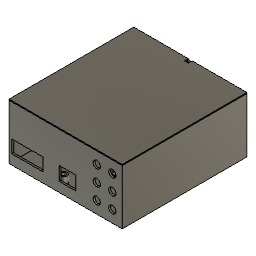
Case (Autodesk Fusion 360 design; units mm, degrees)
Autodesk Fusion 360 part; units mm, degrees
note: some values were not read from the file. Chosen so that the rebuilt part matches the saved one: which bodies a step acts on; which face or edge a step refers to. Set by a fixed rule: which sketch regions a step uses.
sketch "Base" plane through (0, 0, 0) normal (0, 0, 1) x (1, 0, 0) in component "PCB"
  line L0 (58.9, 60.9) -> (0, 60.9)
  line L1 (0, 60.9) -> (0, 0)
  line L2 (0, 0) -> (58.9, 0)
  line L3 (58.9, 0) -> (58.9, 60.9)
  circle A0 centre (3.45, 57.45) radius 1.6
  line L4 (29.45, 60.9) -> (29.45, 0) construction
  line L5 (0, 30.45) -> (58.9, 30.45) construction
  circle A1 centre (55.45, 57.45) radius 1.6
  circle A2 centre (3.45, 3.45) radius 1.6
  circle A3 centre (55.45, 3.45) radius 1.6
  dimension "d1" = 58.9
  dimension "d2" = 60.9
  dimension "d3" = 3.2
  dimension "d4" = 3.45
  dimension "d5" = 3.45
  constraint horizontal L0
  constraint vertical L1
  constraint horizontal L2
  constraint vertical L3
  constraint coincident L1.end L2.start
  constraint midpoint L0 L4.start
  constraint midpoint L2 L4.end
  constraint midpoint L1 L5.start
  constraint midpoint L3 L5.end
  constraint symmetric A0 L4 A1
  constraint symmetric A0 L5 A2
  constraint symmetric L5 A1 A3
  measures "d1" distance of L1.end L2.end
  measures "d2" distance of L0.end L1.end
  measures "d3" diameter of A0
  measures "d4" distance of L0 A0.centre
  measures "d5" distance of L1 A0.centre
extrude "Extrude1" add sketch "Base" along normal blind 24.2 makes body 1 in component "PCB"
sketch "USB port" plane through (0, 60.9, 0) normal (0, 1, 0) x (-1, 0, 0) in component "PCB"
  line L0 (-58.9, 0) -> (0, 0)
  line L1 (0, 0) -> (0, 24.2)
  line L2 (0, 24.2) -> (-58.9, 24.2)
  line L3 (-58.9, 24.2) -> (-58.9, 0)
  line L4 (-44.9, 16.5) -> (-36.9, 16.5)
  line L5 (-36.9, 16.5) -> (-36.9, 13.5)
  line L6 (-36.9, 13.5) -> (-44.9, 13.5)
  line L7 (-44.9, 13.5) -> (-44.9, 16.5)
  dimension "d8" = 8
  dimension "d9" = 3
  dimension "d10" = 14
  dimension "d11" = 13.5
  constraint horizontal L4
  constraint vertical L5
  constraint horizontal L6
  constraint vertical L7
  measures "d8" distance of L4.start L4.end
  measures "d9" distance of L4.start L6.end
  measures "d10" distance of L3 L7
  measures "d11" distance of L0 L6
extrude "Extrude2" add sketch "USB port" along normal blind 1 contours L4 L5 L6 L7 bodies 1 in component "PCB"
sketch "Base (2)" plane through (0, 0, 0) normal (0, 0, 1) x (1, 0, 0) in component "RJ45 breakout"
  line L0 (35.9, 21.4) -> (0, 21.4)
  line L1 (0, 21.4) -> (0, 0)
  line L2 (0, 0) -> (35.9, 0)
  line L3 (35.9, 0) -> (35.9, 21.4)
  circle A0 centre (4, 5) radius 1.6
  line L4 (17.95, 21.4) -> (17.95, 0) construction
  circle A1 centre (31.9, 5) radius 1.6
  dimension "d14" = 35.9
  dimension "d15" = 21.4
  dimension "d16" = 3.2
  dimension "d17" = 5
  dimension "d18" = 4
  constraint horizontal L0
  constraint vertical L1
  constraint horizontal L2
  constraint vertical L3
  constraint coincident L1.end L2.start
  constraint midpoint L0 L4.start
  constraint midpoint L2 L4.end
  constraint symmetric A0 L4 A1
  measures "d14" distance of L0.start L0.end
  measures "d15" distance of L0.end L1.end
  measures "d16" diameter of A0
  measures "d17" distance of L2 A0.centre
  measures "d18" distance of L1 A0.centre
extrude "Extrude1'" add sketch "Base (2)" along normal blind 1.5 separate body makes body 2 in component "RJ45 breakout"
sketch "Port" plane through (0, 0, 1.5) normal (0, 0, 1) x (-1, 0, 0) in component "RJ45 breakout"
  circle A0 centre (-31.9, -5) radius 1.6
  circle A1 centre (-4, -5) radius 1.6
  line L0 (-35.9, 0) -> (-35.9, -21.4)
  line L1 (-35.9, -21.4) -> (0, -21.4)
  line L2 (0, -21.4) -> (0, 0)
  line L3 (0, 0) -> (-35.9, 0)
  line L4 (-9.8, -13.3) -> (-26.1, -13.3)
  line L5 (-26.1, -13.3) -> (-26.1, 2.1)
  line L6 (-26.1, 2.1) -> (-9.8, 2.1)
  line L7 (-9.8, 2.1) -> (-9.8, -13.3)
  dimension "d21" = 16.3
  dimension "d22" = 15.4
  dimension "d23" = 2.1
  dimension "d24" = 35.9
  dimension "d25" = 9.8
  constraint horizontal L4
  constraint vertical L5
  constraint horizontal L6
  constraint vertical L7
  measures "d21" distance of L4.start L4.end
  measures "d22" distance of L4.start L6.end
  measures "d23" distance of L3 L6
  measures "d24" distance of L0.end L1.end
  measures "d25" distance of L2 L7
extrude "Extrude2'" add sketch "Port" along normal blind 13.3 contours L3 L5 L6 L7 | L3 L4 L5 L7 bodies 2 in component "RJ45 breakout"
sketch "Base (3)" plane through (0, 0, 0) normal (0, 0, 1) x (1, 0, 0) in component "UART to RS-232 converter"
  line L0 (31.6, 28) -> (0, 28)
  line L1 (0, 28) -> (0, 0)
  line L2 (0, 0) -> (31.6, 0)
  line L3 (31.6, 0) -> (31.6, 28)
  circle A0 centre (2.1, 25.7) radius 1.6
  line L4 (15.8, 28) -> (15.8, 0) construction
  circle A1 centre (29.5, 25.7) radius 1.6
  dimension "d28" = 28
  dimension "d29" = 31.6
  dimension "d30" = 3.2
  dimension "d31" = 2.1
  dimension "d32" = 2.3
  constraint horizontal L0
  constraint vertical L1
  constraint horizontal L2
  constraint vertical L3
  constraint coincident L1.end L2.start
  constraint midpoint L0 L4.start
  constraint midpoint L2 L4.end
  constraint symmetric A0 L4 A1
  measures "d28" distance of L0.end L1.end
  measures "d29" distance of L0.start L0.end
  measures "d30" diameter of A0
  measures "d31" distance of L1 A0.centre
  measures "d32" distance of L0 A0.centre
extrude "Extrude1''" add sketch "Base (3)" along normal blind 1.5 separate body makes body 3 in component "UART to RS-232 converter"
sketch "Port (2)" plane through (0, 0, 1.5) normal (0, 0, 1) x (-1, 0, 0) in component "UART to RS-232 converter"
  circle A0 centre (-29.5, -25.7) radius 1.6
  circle A1 centre (-2.1, -25.7) radius 1.6
  line L0 (-31.6, 0) -> (-31.6, -28)
  line L1 (-31.6, -28) -> (0, -28)
  line L2 (0, -28) -> (0, 0)
  line L3 (0, 0) -> (-31.6, 0)
  line L4 (0, -12.3) -> (-31.6, -12.3)
  line L5 (-31.6, -12.3) -> (-31.6, 17.9)
  line L6 (-31.6, 17.9) -> (0, 17.9)
  line L7 (0, 17.9) -> (0, -12.3)
  dimension "d35" = 30.2
  dimension "d36" = 12.3
  constraint horizontal L4
  constraint vertical L5
  constraint horizontal L6
  constraint vertical L7
  constraint collinear L2 L7
  constraint collinear L0 L5
  measures "d35" distance of L4.start L6.end
  measures "d36" distance of L3 L4
extrude "Extrude2''" add sketch "Port (2)" along normal blind 12.7 contours L0 L2 L3 L4 L5 L7 | L3 L5 L6 L7 bodies 3 in component "UART to RS-232 converter"
sketch "Sketch1" plane through (0, 0, 0) normal (0, 0, 1) x (1, 0, 0) in component "Relay"
  line L0 (16.35, -19.7) -> (-16.35, -19.7)
  line L1 (-16.35, -19.7) -> (-16.35, 19.7)
  line L2 (-16.35, 19.7) -> (16.35, 19.7)
  line L3 (16.35, 19.7) -> (16.35, -19.7)
  line L4 (16.35, -19.7) -> (-16.35, 19.7) construction
  line L5 (-16.35, -19.7) -> (16.35, 19.7) construction
  dimension "d139" = 32.7
  dimension "d140" = 39.4
  constraint horizontal L0
  constraint perpendicular L0 L1
  constraint parallel L0 L2
  constraint parallel L1 L3
  constraint coincident L4 origin
  constraint coincident L5 origin
  measures "d139" distance of L1.end L2.end
  measures "d140" distance of L0.start L2.end
extrude "Extrude1'''" add sketch "Sketch1" along normal blind 21 separate body makes body 4 in component "Relay"
ref_plane "WorkPlane1" through (0, 0, 10.5) normal (-1, 0, 0) x (0, -1, 0) in component "Relay"
ref_plane "WorkPlane2" through (0, 0, 10.5) normal (0, -1, 0) x (1, 0, 0) in component "Relay"
sketch "Sketch2" plane through (0, 0, 21) normal (0, 0, 1) x (-1, 0, 0) in component "Relay"
  line L0 (-16.35, -19.7) -> (16.35, -19.7)
  line L1 (16.35, -19.7) -> (16.35, 19.7)
  line L2 (16.35, 19.7) -> (-16.35, 19.7)
  line L3 (-16.35, 19.7) -> (-16.35, -19.7)
  circle A0 centre (12.55, -15.7) radius 1.5
  line L4 (0, -23.64) -> (0, 23.64)
  circle A1 centre (-12.55, -15.7) radius 1.5
  line L5 (19.62, 0) -> (-19.62, 0)
  circle A2 centre (12.55, 15.7) radius 1.5
  circle A3 centre (-12.55, 15.7) radius 1.5
  dimension "d143" = 3
  dimension "d144" = 4
  dimension "d145" = 3.8
  constraint symmetric A0 L4 A1
  constraint symmetric A0 L5 A2
  constraint symmetric A1 L5 A3
  measures "d143" diameter of A0
  measures "d144" distance of L0 A0.centre
  measures "d145" distance of L1 A0.centre
extrude "Extrude2'''" cut sketch "Sketch2" against normal up to surface (21 mm away) contours A0 | A1 | A2 | A3 bodies 4 in component "Relay"
sketch "Sketch1 (2)" plane through (0, 0, 0) normal (0, 1, 0) x (1, 0, 0) in component "Banana socket"
  circle A0 centre (0, 0) radius 6
  dimension "d148" = 12
  constraint coincident A0.centre origin
  measures "d148" diameter of A0
extrude "Extrude1''''" add sketch "Sketch1 (2)" along normal blind 24 separate body makes body 5 in component "Banana socket"
sketch "Sketch2 (2)" plane through (0, 24, 0) normal (0, 1, 0) x (-1, 0, 0) in component "Banana socket"
  circle A0 centre (0, 0) radius 6
  circle A1 centre (0, 0) radius 3.8
  dimension "d151" = 7.6
  constraint coincident A0.centre A1.centre
  measures "d151" diameter of A1
extrude "Extrude2''''" add sketch "Sketch2 (2)" along normal blind 21.5 contours A1 bodies 5 in component "Banana socket"
other "GeometricRelationship15"
other "GeometricRelationship18"
other "GeometricRelationship19"
pattern_linear "00000000-0000-0000-0000-000000000000" [suppressed]
sketch "Sketch10" plane through (0, 0, 0) normal (0, 0, 1) x (1, 0, 0) in component "Case"
  circle A0 centre (8.2, 75.65) radius 1.6
  circle A1 centre (60.2, 75.65) radius 1.6
  circle A2 centre (60.2, 21.65) radius 1.6
  circle A3 centre (8.2, 21.65) radius 1.6
  circle A4 centre (6.85, -7.6) radius 1.6
  circle A5 centre (34.25, -7.6) radius 1.6
  circle A6 centre (77.45, 15.7) radius 1.5
  circle A7 centre (102.55, 15.7) radius 1.5
  circle A8 centre (102.55, -15.7) radius 1.5
  circle A9 centre (77.45, -15.7) radius 1.5
  circle A10 centre (77.45, 65.1) radius 1.5
  circle A11 centre (102.55, 65.1) radius 1.5
  circle A12 centre (77.45, 33.7) radius 1.5
  circle A13 centre (102.55, 33.7) radius 1.5
  circle A14 centre (50.35, -44.1) radius 1.6
  circle A15 centre (78.25, -44.1) radius 1.6
  circle A16 centre (34.25, -7.6) radius 1.6
  circle A17 centre (6.85, -7.6) radius 1.6
  line L0 (36.35, -5.3) -> (36.35, -33.3)
  line L1 (36.35, -33.3) -> (4.75, -33.3)
  line L2 (4.75, -33.3) -> (4.75, -5.3)
  line L3 (4.75, -5.3) -> (36.35, -5.3)
  circle A18 centre (8.2, 75.65) radius 2
  circle A19 centre (8.2, 75.65) radius 3.5
  circle A20 centre (60.2, 75.65) radius 2
  circle A21 centre (60.2, 75.65) radius 3.5
  circle A22 centre (8.2, 21.65) radius 2
  circle A23 centre (8.2, 21.65) radius 3.5
  circle A24 centre (60.2, 21.65) radius 2
  circle A25 centre (60.2, 21.65) radius 3.5
  circle A26 centre (77.45, 65.1) radius 2
  circle A27 centre (77.45, 65.1) radius 3.5
  circle A28 centre (102.55, 65.1) radius 2
  circle A29 centre (102.55, 65.1) radius 3.5
  circle A30 centre (102.55, 33.7) radius 2
  circle A31 centre (102.55, 33.7) radius 3.5
  circle A32 centre (77.45, 33.7) radius 2
  circle A33 centre (77.45, 33.7) radius 3.5
  circle A34 centre (77.45, 15.7) radius 2
  circle A35 centre (77.45, 15.7) radius 3.5
  circle A36 centre (102.55, 15.7) radius 2
  circle A37 centre (102.55, 15.7) radius 3.5
  circle A38 centre (102.55, -15.7) radius 2
  circle A39 centre (102.55, -15.7) radius 3.5
  circle A40 centre (77.45, -15.7) radius 2
  circle A41 centre (77.45, -15.7) radius 3.5
  circle A42 centre (6.85, -7.6) radius 2
  circle A43 centre (6.85, -7.6) radius 3.5
  circle A44 centre (34.25, -7.6) radius 2
  circle A45 centre (34.25, -7.6) radius 3.5
  circle A46 centre (50.35, -44.1) radius 2
  circle A47 centre (50.35, -44.1) radius 3.5
  circle A48 centre (78.25, -44.1) radius 2
  circle A49 centre (78.25, -44.1) radius 3.5
  circle A50 centre (20.55, -30.8) radius 2.5
  point P0 (20.55, -33.3)
  dimension "d219" = 4
  dimension "d220" = 7
  dimension "d221" = 4
  dimension "d222" = 7
  dimension "d223" = 4
  dimension "d224" = 7
  dimension "d225" = 4
  dimension "d226" = 7
  dimension "d227" = 4
  dimension "d228" = 7
  dimension "d229" = 4
  dimension "d230" = 7
  dimension "d231" = 4
  dimension "d232" = 7
  dimension "d233" = 4
  dimension "d234" = 7
  dimension "d235" = 4
  dimension "d236" = 7
  dimension "d237" = 4
  dimension "d238" = 7
  dimension "d239" = 4
  dimension "d240" = 7
  dimension "d241" = 4
  dimension "d242" = 7
  dimension "d243" = 4
  dimension "d244" = 7
  dimension "d245" = 4
  dimension "d246" = 7
  dimension "d247" = 4
  dimension "d248" = 7
  dimension "d249" = 4
  dimension "d250" = 7
  dimension "d251" = 5
  constraint coincident A0.centre A18.centre
  constraint coincident A1.centre A20.centre
  constraint coincident A3.centre A22.centre
  constraint coincident A2.centre A24.centre
  constraint coincident A10.centre A26.centre
  constraint coincident A11.centre A28.centre
  constraint coincident A13.centre A30.centre
  constraint coincident A12.centre A32.centre
  constraint coincident A6.centre A34.centre
  constraint coincident A7.centre A36.centre
  constraint coincident A8.centre A38.centre
  constraint coincident A9.centre A40.centre
  constraint coincident A4.centre A17.centre
  constraint coincident A5.centre A16.centre
  constraint coincident A14.centre A46.centre
  constraint coincident A15.centre A48.centre
  constraint midpoint L1 P0
  constraint vertical A50.centre P0
  constraint tangent L1 A50
  measures "d219" diameter of A18
  measures "d220" diameter of A19
  measures "d221" diameter of A20
  measures "d222" diameter of A21
  measures "d223" diameter of A22
  measures "d224" diameter of A23
  measures "d225" diameter of A24
  measures "d226" diameter of A25
  measures "d227" diameter of A26
  measures "d228" diameter of A27
  measures "d229" diameter of A28
  measures "d230" diameter of A29
  measures "d231" diameter of A30
  measures "d232" diameter of A31
  measures "d233" diameter of A32
  measures "d234" diameter of A33
  measures "d235" diameter of A34
  measures "d236" diameter of A35
  measures "d237" diameter of A36
  measures "d238" diameter of A37
  measures "d239" diameter of A38
  measures "d240" diameter of A39
  measures "d241" diameter of A40
  measures "d242" diameter of A41
  measures "d243" diameter of A42
  measures "d244" diameter of A43
  measures "d245" diameter of A44
  measures "d246" diameter of A45
  measures "d247" diameter of A46
  measures "d248" diameter of A47
  measures "d249" diameter of A48
  measures "d250" diameter of A49
  measures "d251" diameter of A50
extrude "Extrude10" add sketch "Sketch10" against normal blind 8 separate body contours L0 L3 A45 | L0 L3 A45 | A50 | L2 L3 A43 | L2 L3 A43 | A19 | A21 | A23 | A25 | A27 | A29 | A31 | A33 | A35 | A37 | A39 | A41 | A47 | A49 makes body 6 at (23.0469, -30.9246, -5.3333) makes body 7 at (106.0456, -15.8745, -5.3333) makes body 8 at (106.0456, 33.5255, -5.3333) makes body 9 at (11.6956, 21.4755, -5.3333) makes body 10 at (57.2135, 73.825, -5.3333) makes body 11 at (100.1062, 62.5945, -5.3333) makes body 12 at (101.4353, 12.3823, -5.3333) makes body 13 at (37.7326, -7.2515, -2.6667) makes body 14 at (53.8456, -44.2745, -5.3333) makes body 15 at (76.3353, -19.0177, -5.3333) makes body 16 at (80.1312, 35.9498, -5.3333) makes body 17 at (63.6956, 21.4755, -5.3333) makes body 18 at (5.2135, 73.825, -5.3333) makes body 19 at (80.9456, 64.9255, -5.3333) makes body 20 at (80.9456, 15.5255, -5.3333) makes body 21 at (10.3456, -7.7745, -5.3333) makes body 22 at (75.8062, -46.6055, -5.3333) in component "Case"
sketch "Sketch11" plane through (0, 0, -8) normal (0, 0, -1) x (1, 0, 0) in component "Case"
  circle A0 centre (34.25, 7.6) radius 2
  circle A1 centre (34.25, 7.6) radius 3.5
  circle A2 centre (8.2, -75.65) radius 1.6
  circle A3 centre (8.2, -21.65) radius 1.6
  circle A4 centre (60.2, -21.65) radius 1.6
  circle A5 centre (60.2, -75.65) radius 1.6
  line L0 (63.65, -79.1) -> (63.65, -18.2)
  line L1 (63.65, -18.2) -> (4.75, -18.2)
  line L2 (4.75, -18.2) -> (4.75, -79.1)
  line L3 (4.75, -79.1) -> (63.65, -79.1)
  line L4 (109.45, 32.7) -> (117.05, 32.7)
  line L5 (117.05, 54.2) -> (109.45, 54.2)
  line L6 (2.35, 52.2) -> (122.05, 52.2)
  line L7 (122.05, 52.2) -> (122.05, -80.1)
  line L8 (122.05, -80.1) -> (2.35, -80.1)
  line L9 (2.35, -80.1) -> (2.35, 52.2)
  circle A6 centre (6.85, 7.6) radius 3.5
  line L10 (56.15, 51.2) -> (72.45, 51.2)
  line L11 (72.45, 51.2) -> (72.45, 35.8)
  line L12 (72.45, 35.8) -> (56.15, 35.8)
  line L13 (56.15, 35.8) -> (56.15, 51.2)
  dimension "d255" = 1
  dimension "d256" = 5
  dimension "d257" = 4.5
  dimension "d258" = 7
  dimension "d264" = 1
  constraint horizontal L6
  constraint vertical L7
  constraint horizontal L8
  constraint vertical L9
  measures "d255" distance of L3 L8
  measures "d256" distance of L4.end L7
  measures "d257" distance of L9 A6.centre
  measures "d258" diameter of A6
  measures "d264" distance of L6 L10
extrude "Extrude11" add sketch "Sketch11" along normal blind 2 contours A0 | A1 | A2 | A3 | A4 | A5 | L0 L1 L2 L3 | L6 L7 L8 L9 | A6 | L10 L11 L12 L13 bodies 6 7 8 9 10 11 12 13 14 15 16 17 18 19 20 21 22 in component "Case"
sketch "Sketch12" plane through (0, 0, -10) normal (0, 0, -1) x (1, 0, 0) in component "Case"
  line L0 (2.35, -80.1) -> (122.05, -80.1)
  line L1 (122.05, -80.1) -> (122.05, 52.2)
  line L2 (122.05, 52.2) -> (2.35, 52.2)
  line L3 (2.35, 52.2) -> (2.35, -80.1)
  line L4 (0.35, -82.1) -> (124.05, -82.1)
  line L5 (124.05, -82.1) -> (124.05, 54.2)
  line L6 (124.05, 54.2) -> (0.35, 54.2)
  line L7 (0.35, 54.2) -> (0.35, -82.1)
  dimension "d261" = 2
extrude "Extrude12" add sketch "Sketch12" against normal blind 60 bodies 6 in component "Case"
sketch "Sketch13" plane through (0, 82.1, 0) normal (0, 1, 0) x (-1, 0, 0) in component "Case"
  line L0 (-124.05, -10) -> (-0.35, -10)
  line L1 (-0.35, -10) -> (-0.35, 50)
  line L2 (-0.35, 50) -> (-124.05, 50)
  line L3 (-124.05, 50) -> (-124.05, -10)
  line L4 (-49.65, 13.5) -> (-41.65, 13.5)
  line L5 (-41.65, 13.5) -> (-41.65, 16.5)
  line L6 (-41.65, 16.5) -> (-49.65, 16.5)
  line L7 (-49.65, 16.5) -> (-49.65, 13.5)
  line L8 (-51.65, 19.5) -> (-39.65, 19.5)
  line L9 (-39.65, 19.5) -> (-39.65, 10.5)
  line L10 (-39.65, 10.5) -> (-51.65, 10.5)
  line L11 (-51.65, 10.5) -> (-51.65, 19.5)
  dimension "d265" = 12
  dimension "d266" = 9
  dimension "d267" = 3
  dimension "d268" = 8
  dimension "d269" = 2
  dimension "d270" = 3
  constraint horizontal L8
  constraint vertical L9
  constraint horizontal L10
  constraint vertical L11
  measures "d265" distance of L8.start L8.end
  measures "d266" distance of L8.end L9.end
  measures "d267" distance of L4.start L6.end
  measures "d268" distance of L4.start L4.end
  measures "d269" distance of L7 L11
  measures "d270" distance of L6 L8
extrude "Extrude13" cut sketch "Sketch13" against normal up to surface (2 mm away) contours L4 L5 L6 L7 | L8 L9 L10 L11 bodies 6 in component "Case"
sketch "Sketch14" plane through (0, -54.2, 0) normal (0, -1, 0) x (1, 0, 0) in component "Case"
  line L0 (0.35, -10) -> (124.05, -10)
  line L1 (124.05, -10) -> (124.05, 50)
  line L2 (124.05, 50) -> (0.35, 50)
  line L3 (0.35, 50) -> (0.35, -10)
  line L4 (4.75, 1.5) -> (36.35, 1.5)
  line L5 (36.35, 1.5) -> (36.35, 14.2)
  line L6 (36.35, 14.2) -> (4.75, 14.2)
  line L7 (4.75, 14.2) -> (4.75, 1.5)
  line L8 (56.15, 1.5) -> (72.45, 1.5)
  line L9 (72.45, 1.5) -> (72.45, 14.8)
  line L10 (72.45, 14.8) -> (56.15, 14.8)
  line L11 (56.15, 14.8) -> (56.15, 1.5)
  circle A0 centre (96.25, 37) radius 3.8
  circle A1 centre (113.25, 37) radius 3.8
  circle A2 centre (96.25, 20) radius 3.8
  circle A3 centre (113.25, 20) radius 3.8
  circle A4 centre (96.25, 3) radius 3.8
  circle A5 centre (113.25, 3) radius 3.8
  line L12 (3.55, 14.85) -> (37.55, 14.85)
  line L13 (37.55, 14.85) -> (37.55, 0.85)
  line L14 (37.55, 0.85) -> (3.55, 0.85)
  line L15 (3.55, 0.85) -> (3.55, 14.85)
  line L16 (55.3, 15.65) -> (73.3, 15.65)
  line L17 (73.3, 15.65) -> (73.3, 0.65)
  line L18 (73.3, 0.65) -> (55.3, 0.65)
  line L19 (55.3, 0.65) -> (55.3, 15.65)
  circle A6 centre (96.25, 37) radius 4
  circle A7 centre (113.25, 37) radius 4
  circle A8 centre (96.25, 20) radius 4
  circle A9 centre (113.25, 20) radius 4
  circle A10 centre (96.25, 3) radius 4
  circle A11 centre (113.25, 3) radius 4
  dimension "d273" = 34
  dimension "d274" = 14
  dimension "d275" = 31.6
  dimension "d276" = 12.7
  dimension "d277" = 1.2
  dimension "d278" = 0.65
  dimension "d279" = 18
  dimension "d280" = 15
  dimension "d281" = 13.3
  dimension "d282" = 16.3
  dimension "d283" = 0.85
  dimension "d284" = 0.85
  dimension "d285" = 8
  dimension "d286" = 8
  dimension "d287" = 8
  dimension "d288" = 8
  dimension "d289" = 8
  dimension "d290" = 8
  constraint horizontal L12
  constraint vertical L13
  constraint horizontal L14
  constraint vertical L15
  constraint horizontal L16
  constraint vertical L17
  constraint horizontal L18
  constraint vertical L19
  constraint coincident A0.centre A6.centre
  constraint coincident A1.centre A7.centre
  constraint coincident A2.centre A8.centre
  constraint coincident A3.centre A9.centre
  constraint coincident A4.centre A10.centre
  constraint coincident A5.centre A11.centre
  measures "d273" distance of L12.start L12.end
  measures "d274" distance of L12.end L13.end
  measures "d275" distance of L5.end L6.end
  measures "d276" distance of L4.start L6.end
  measures "d277" distance of L7 L15
  measures "d278" distance of L6 L12
  measures "d279" distance of L16.start L16.end
  measures "d280" distance of L16.start L18.end
  measures "d281" distance of L8.end L9.end
  measures "d282" distance of L8.start L8.end
  measures "d283" distance of L11 L19
  measures "d284" distance of L10 L16
  measures "d285" diameter of A6
  measures "d286" diameter of A7
  measures "d287" diameter of A8
  measures "d288" diameter of A9
  measures "d289" diameter of A10
  measures "d290" diameter of A11
extrude "Extrude14" cut sketch "Sketch14" against normal up to surface (2 mm away) contours L4 L5 L6 L7 | L8 L9 L10 L11 | A0 | A1 | A2 | A3 | A4 | A5 | L12 L13 L14 L15 | L16 L17 L18 L19 | A6 | A7 | A8 | A9 | A10 | A11 bodies 6 in component "Case"
sketch "Sketch15" plane through (0, 0, 50) normal (0, 0, 1) x (-1, 0, 0) in component "Case"
  line L0 (-2.35, 52.2) -> (-2.35, -80.1)
  line L1 (-2.35, -80.1) -> (-122.05, -80.1)
  line L2 (-122.05, -80.1) -> (-122.05, 52.2)
  line L3 (-122.05, 52.2) -> (-2.35, 52.2)
  line L4 (-0.35, -82.1) -> (-0.35, 54.2)
  line L5 (-0.35, 54.2) -> (-124.05, 54.2)
  line L6 (-124.05, 54.2) -> (-124.05, -82.1)
  line L7 (-124.05, -82.1) -> (-0.35, -82.1)
  line L8 (-121.95, 52.1) -> (-2.45, 52.1)
  line L9 (-2.45, 52.1) -> (-2.45, -80)
  line L10 (-2.45, -80) -> (-121.95, -80)
  line L11 (-121.95, -80) -> (-121.95, 52.1)
  dimension "d293" = 0.1
extrude "Extrude15" add sketch "Sketch15" against normal blind 1 separate body contours L8 L9 L10 L11 makes body 23 in component "Case"
sketch "Sketch16" plane through (0, 0, 50) normal (0, 0, 1) x (-1, 0, 0) in component "Case"
  line L0 (-121.95, -80) -> (-2.45, -80)
  line L1 (-2.45, -80) -> (-2.45, 52.1)
  line L2 (-2.45, 52.1) -> (-121.95, 52.1)
  line L3 (-121.95, 52.1) -> (-121.95, -80)
  line L4 (-124.05, -82.1) -> (-0.35, -82.1)
  line L5 (-2.35, 52.2) -> (-2.35, -80.1)
  line L6 (-2.35, -80.1) -> (-122.05, -80.1)
  line L7 (-122.05, -80.1) -> (-122.05, 52.2)
  line L8 (-122.05, 52.2) -> (-2.35, 52.2)
  line L9 (-0.35, -82.1) -> (-0.35, 54.2)
  line L10 (-0.35, 54.2) -> (-124.05, 54.2)
  line L11 (-124.05, 54.2) -> (-124.05, -82.1)
  line L12 (-124.05, -82.1) -> (-0.35, -82.1)
extrude "Extrude16" add sketch "Sketch16" along normal blind 1 separate body contours L0 L1 L2 L3 | L4 L9 L10 L11 L12 | L5 L6 L7 L8 makes body 24 in component "Case"
combine "Combine2" operation add target body 23 tool bodies 24 in component "Case"
sketch "Sketch17" plane through (0, 0, 49) normal (0, 0, -1) x (1, 0, 0) in component "Case"
  line L0 (2.45, -80) -> (121.95, -80)
  line L1 (121.95, -80) -> (121.95, 52.1)
  line L2 (121.95, 52.1) -> (2.45, 52.1)
  line L3 (2.45, 52.1) -> (2.45, -80)
  line L4 (64.2, -80) -> (60.2, -80)
  line L5 (60.2, -80) -> (60.2, -78)
  line L6 (60.2, -78) -> (64.2, -78)
  line L7 (64.2, -78) -> (64.2, -80)
  line L8 (64.2, -80) -> (60.2, -78) construction
  line L9 (60.2, -80) -> (64.2, -78) construction
  point P0 (62.2, -79)
  point P1 (62.2, -80)
  dimension "d298" = 4
  dimension "d299" = 2
  constraint horizontal L4
  constraint perpendicular L4 L5
  constraint parallel L4 L6
  constraint parallel L5 L7
  constraint coincident L8 P0
  constraint coincident L9 P0
  constraint midpoint L0 P1
  constraint vertical P0 P1
  constraint collinear L0 L4
  measures "d298" distance of L5.end L6.end
  measures "d299" distance of L4.end L5.end
extrude "Extrude17" cut sketch "Sketch17" against normal up to surface (2 mm away) contours L0 L4 L5 L6 L7 bodies 23 in component "Case"
sketch "Sketch18" plane through (0, 0, 51) normal (0, 0, 1) x (-1, 0, 0) in component "Case"
  line L0 (-64.2, -80) -> (-64.2, -78)
  line L1 (-64.2, -78) -> (-60.2, -78)
  line L2 (-60.2, -78) -> (-60.2, -80)
  line L3 (-60.2, -80) -> (-64.2, -80)
  line L4 (-124.05, -82.1) -> (-0.35, -82.1)
  line L5 (-0.35, -82.1) -> (-0.35, 54.2)
  line L6 (-0.35, 54.2) -> (-124.05, 54.2)
  line L7 (-124.05, 54.2) -> (-124.05, -82.1)
  line L8 (-64.2, -80) -> (-64.2, -82.1)
  line L9 (-60.2, -80) -> (-60.2, -82.1)
  line L10 (-64.2, -82.1) -> (-60.2, -82.1)
  line L11 (-64.2, -80) -> (-60.2, -80)
  constraint coincident L0.start L3.end
  constraint coincident L4 L8.end
  constraint perpendicular L4 L8
  constraint coincident L2.end L3.start
  constraint coincident L4 L9.end
  constraint perpendicular L4 L9
extrude "Extrude18" cut sketch "Sketch18" against normal up to surface (1 mm away) contours L3 L4 L8 L9 L10 L11 bodies 23 in component "Case"
component "PCB" placed x (1, 0, 0) y (0, 1, 0) z (0, 0, 1) at (4.75, 18.2, 0)
component "RJ45 breakout" placed x (1, 0, 0) y (0, 1, 0) z (0, 0, 1) at (46.35, -49.1, 0)
component "UART to RS-232 converter" placed x (1, 0, 0) y (0, 1, 0) z (0, 0, 1) at (4.75, -33.3, 0)
component "Relay" placed x (1, 0, 0) y (0, 1, 0) z (0, 0, 1) at (90, 49.4, 0)
component "Relay" placed x (1, 0, 0) y (0, 1, 0) z (0, 0, 1) at (90, 0, 0)
component "Banana socket" placed x (1, 0, 0) y (0, 1, 0) z (0, 0, 1) at (96.25, -78.2, 3)
component "Case" placed x (1, 0, 0) y (0, 1, 0) z (0, 0, 1) at (0, 0, 0)
component "Banana socket" placed x (1, 0, 0) y (0, 1, 0) z (0, 0, 1) at (96.25, -78.2, 20)
component "Banana socket" placed x (1, 0, 0) y (0, 1, 0) z (0, 0, 1) at (96.25, -78.2, 37)
component "Banana socket" placed x (1, 0, 0) y (0, 1, 0) z (0, 0, 1) at (113.25, -78.2, 3)
component "Banana socket" placed x (1, 0, 0) y (0, 1, 0) z (0, 0, 1) at (113.25, -78.2, 20)
component "Banana socket" placed x (1, 0, 0) y (0, 1, 0) z (0, 0, 1) at (113.25, -78.2, 37)
equation "d4 = 1.85 mm + d3 / 2"
equation "d5 = d4"
equation "d17 = 3.4 mm + d16 / 2"
equation "d18 = 2.4 mm + d16 / 2"
equation "d25 = ( d24 - d21 ) / 2"
equation "d31 = 0.5 mm + d30 / 2"
equation "d32 = 0.7 mm + d30 / 2"
equation "d144 = 2.5 mm + d143 / 2"
equation "d145 = 2.3 mm + d143 / 2"
equation "d257 = d258 / 2 + 1 mm"
equation "d269 = ( d265 - d268 ) / 2"
equation "d270 = ( d266 - d267 ) / 2"
equation "d277 = ( d273 - d275 ) / 2"
equation "d278 = ( d274 - d276 ) / 2"
equation "d283 = ( d279 - d282 ) / 2"
equation "d284 = ( d280 - d281 ) / 2"
named bodies: "Body", "Lid"
